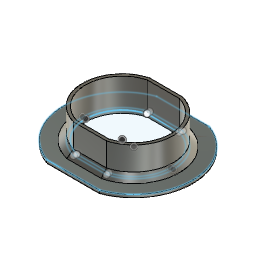
TubeWithSkirt v2 (Autodesk Fusion 360 design; units mm, degrees)
Autodesk Fusion 360 part; units mm, degrees
sketch "Sketch1" plane through (0, 0, 0) normal (0, 0, 1) x (1, 0, 0)
  line L0 (33.0292, 88.6269) -> (55.0292, 88.6269)
  line L1 (33.0292, 40.6269) -> (55.0292, 40.6269)
  arc A0 (33.0292, 88.6269) -> (33.0292, 40.6269) centre (40.0292, 64.6269) ccw
  arc A1 (55.0292, 40.6269) -> (55.0292, 88.6269) centre (48.0292, 64.6269) ccw
  arc A2 (55.3093, 38.6269) -> (55.3093, 90.6269) centre (48.0292, 64.6269) ccw
  line L2 (32.7491, 38.6269) -> (55.3093, 38.6269)
  line L3 (32.7491, 90.6269) -> (55.3093, 90.6269)
  arc A3 (32.7491, 90.6269) -> (32.7491, 38.6269) centre (40.0292, 64.6269) ccw
  arc A4 (33.0292, 88.6269) -> (33.0292, 40.6269) centre (40.0292, 64.6269) ccw
  arc A5 (26.1098, 102.1269) -> (26.1098, 27.1269) centre (40.0292, 64.6269) ccw
  arc A6 (61.9486, 27.1269) -> (61.9486, 102.1269) centre (48.0292, 64.6269) ccw
  line L4 (26.1098, 102.1269) -> (61.9486, 102.1269)
  line L5 (26.1098, 27.1269) -> (61.9486, 27.1269)
  point P0 (15.0292, 64.6269)
  point P1 (73.0292, 64.6269)
  point P2 (75.0292, 64.6269)
  point P3 (13.0292, 64.6269)
  dimension "d5" = 50
  dimension "d6" = 48
  dimension "d10" = 58
  dimension "d23" = 52
  dimension "d24" = 62
  dimension "d25" = 27
  dimension "d26" = 27
  dimension "d27" = 8
  dimension "d28" = 8
  dimension "d31" = 50
  dimension "d32" = 48
  dimension "d33" = 75
  dimension "d34" = 40
  dimension "d35" = 75
  dimension "d36" = 40
  dimension "d37" = 8
  constraint vertical L0.end L1.end
  constraint coincident L0.start A0.start
  constraint coincident L0.end A1.end
  constraint coincident L1.start A0.end
  constraint coincident L1.end A1.start
  constraint parallel L0 L1
  constraint horizontal L0
  constraint coincident P0 A0
  constraint horizontal A0.centre P0
  constraint horizontal P0 P1
  constraint coincident P1 A1
  constraint vertical A2.end A2.start
  constraint coincident L3.start A3.start
  constraint coincident A2.end L3.end
  constraint coincident L2.start A3.end
  constraint coincident A2.start L2.end
  constraint parallel L2 L3
  constraint horizontal L3
  constraint coincident P3 A3
  constraint horizontal A0.centre P3
  constraint horizontal P2 P3
  constraint coincident P2 A2
  constraint coincident A0.centre A3.centre
  constraint vertical A5.end A5.start
  constraint parallel L4 L5
  constraint horizontal A0.centre A1.centre
  constraint coincident A1.centre A2.centre
  measures "d5" diameter of A0
  measures "d6" distance of L1.start L0.start
  measures "d10" distance of P0 P1
  measures "d23" distance of L2.start L3.start
  measures "d24" distance of P2 P3
  measures "d25" distance of A1.centre A2.end
  measures "d26" distance of L3.start A0.centre
  measures "d27" distance of A0.centre A1.centre
  measures "d28" distance of A1.centre A0.centre
  measures "d31" diameter of A4
  measures "d32" distance of L1.start L0.start
  measures "d33" distance of A5.end A5.start
  measures "d34" distance of A0.centre A5.start
  measures "d35" distance of A6.start A6.end
  measures "d36" distance of A1.centre A6.start
  measures "d37" horizontal distance of A0.centre A1.centre
extrude "Extrude1" add sketch "Sketch1" along normal blind 20 contours A2 L2 L3 A3
extrude "Extrude2" add sketch "Sketch1" against normal blind 2 contours A2 L2 L3 A3 | A5 A6 L4 L5
chamfer "Chamfer1" distance 4 angle 45 4 edges at (44.0292, 90.6269, 0) (13.0292, 64.6269, 0) (75.0292, 64.6269, 0) (44.0292, 38.6269, 0)
